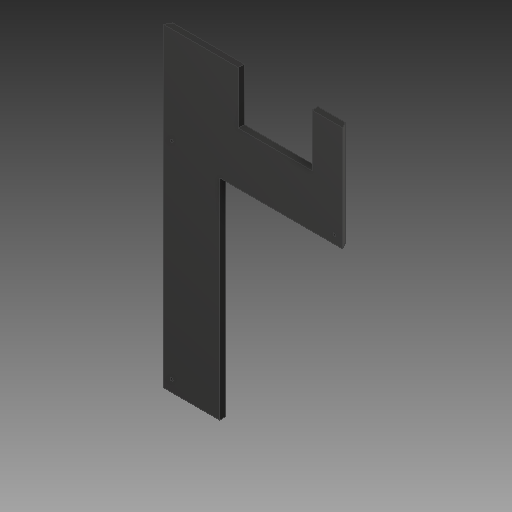
# Autodesk Inventor part: BA03
Saved by Autodesk Inventor 2017 (Build 210142000, 142)
## iProperties
Created: 2018-10-18
Part Number: BA03
Material: ABS Plastic
Document SubType Name: Modeling
Designer: Dell
Density: 1.06 g/cm^3
Appearance: Smooth - Black
Author: Dell
Autodesk Inventor part; units mm, degrees
ref_plane "YZ Plane" through (0, 0, 0) normal (1, 0, 0) x (0, 1, 0)
ref_plane "XZ Plane" through (0, 0, 0) normal (0, 1, 0) x (-1, 0, 0)
ref_plane "XY Plane" through (0, 0, 0) normal (0, 0, 1) x (1, 0, 0)
sketch "Sketch1" plane through (0, 0, 0) normal (0, 0, 1) x (1, 0, 0)
  line L0 (0, 0) -> (292.1, 0)
  line L1 (292.1, 0) -> (292.1, -177.8)
  line L2 (292.1, -177.8) -> (0, -177.8)
  line L3 (0, -177.8) -> (0, 0)
  dimension "d0" = 292.1
  dimension "d1" = 177.8
  constraints: 8 end point, 2 parallel, 1 horizontal, 1 perpendicular
  measures "d0" distance of L1.end L2.end
  measures "d1" distance of L0.end L1.end
extrude "Extrusion1" add sketch "Sketch1" along normal blind 10
sketch "Sketch2" plane through (0, 0, 0) normal (0, 1, 0) x (1, 0, 0)
  line L0 (292.1, -10) -> (0, -10) projected
  line L1 (0, -10) -> (-5.7735, -10)
  line L2 (-5.7735, -10) -> (0, 0)
  line L3 (0, 0) -> (0, -10) projected
  line L4 (0, 0) -> (0, -10) projected
  line L5 (0, -10) -> (0, 0)
  line L6 (292.1, -10) -> (297.8735, -10)
  line L7 (292.1, 0) -> (292.1, -10) projected
  line L8 (297.8735, -10) -> (292.1, 0)
  line L9 (292.1, 0) -> (292.1, -10)
  dimension "d4" = 30
  dimension "d5" = 60
  constraints: 12 end point, 2 collinear, 2 horizontal
  measures "d4" angle of L3 L2
  measures "d5" angle of L6 L8
extrude "Extrusion2" add sketch "Sketch2" against normal blind 177.8
sketch "Sketch3" plane through (0, 0, 10) normal (0, 0, 1) x (1, 0, 0)
  line L0 (46.05, -88.9) -> (246.05, -88.9)
  line L1 (246.05, -88.9) -> (246.05, 0)
  line L2 (246.05, 0) -> (46.05, 0)
  line L3 (46.05, 0) -> (46.05, -88.9)
  line L4 (-5.7735, 0) -> (297.8735, 0) projected
  line L5 (46.05, -88.9) -> (190.7027, -88.9)
  line L6 (121.05, 0) -> (46.05, 0)
  line L7 (46.05, 0) -> (46.05, -88.9)
  line L8 (246.05, 0) -> (171.05, 0)
  line L9 (121.05, -88.9) -> (246.05, -88.9)
  line L10 (246.05, -88.9) -> (246.05, 0)
  line L11 (46.05, 0) -> (121.05, 0)
  line L12 (121.05, 0) -> (121.05, -88.9)
  line L13 (121.05, -88.9) -> (46.05, -88.9)
  line L14 (46.05, -88.9) -> (46.05, 0)
  line L15 (246.05, 0) -> (246.05, 0)
  line L16 (246.05, 0) -> (246.05, -88.9)
  line L17 (246.05, -88.9) -> (246.05, -88.9)
  line L18 (246.05, -88.9) -> (246.05, 0)
  point P0 (0, 0)
  point P1 (146.05, 0)
  point P2 (246.05, -44.45)
  dimension "d8" = 200
  dimension "d9" = 88.9
  dimension "d14" = 75
  constraints: 36 end point, 7 parallel, 5 horizontal, 4 midpoint, 3 perpendicular, 3 point on line, 1 collinear
  measures "d8" distance of L1.end L2.end
  measures "d9" distance of L0.end L1.end
  measures "d14" distance between parallel lines of L3 L12
extrude "Extrusion3" cut sketch "Sketch3" against normal through all contours L12 L2 L1 L0
sketch "Sketch4" plane through (0, 0, 10) normal (0, 0, 1) x (1, 0, 0)
  line L0 (8.1265, -163.9) -> (283.9735, -163.9) construction
  line L1 (297.8735, -177.8) -> (-5.7735, -177.8) construction
  line L2 (297.8735, 0) -> (297.8735, -177.8) construction
  line L3 (-5.7735, 0) -> (-5.7735, -177.8) construction
  circle A0 centre (8.1265, -163.9) radius 2.5
  circle A1 centre (283.9735, -163.9) radius 2.5
  point P0 (0, 0)
  dimension "d16" = 13.9
  dimension "d17" = 13.9
  dimension "d18" = 13.9
  dimension "d19" = 5
  dimension "d20" = 5
  constraints: 2 centre point, 2 coincident, 2 end point, 1 horizontal
  measures "d16" distance between parallel lines of L1 L0
  measures "d17" distance from line of L2 L0.end
  measures "d18" distance from line of L3 L0.start
  measures "d19" diameter of A0
  measures "d20" diameter of A1
extrude "Extrusion4" cut sketch "Sketch4" against normal through all
sketch "Sketch5" plane through (0, 0, 10) normal (0, 0, 1) x (1, 0, 0)
  line L0 (297.8735, -177.8) -> (-5.7735, -177.8) projected
  line L1 (-5.7735, -177.8) -> (89.4765, -177.8)
  line L2 (89.4765, -177.8) -> (89.4765, -533.4)
  line L3 (89.4765, -533.4) -> (-5.7735, -533.4)
  line L4 (-5.7735, -533.4) -> (-5.7735, -177.8)
  point P0 (0, 0)
  dimension "d23" = 95.25
  dimension "d24" = 355.6
  constraints: 8 end point, 2 parallel, 1 horizontal, 1 perpendicular
  measures "d23" distance between parallel lines of L2 L4
  measures "d24" distance of L3.end L0.end
extrude "Extrusion5" add sketch "Sketch5" against normal blind 10
sketch "Sketch6" plane through (-5.7735, -177.8, 0) normal (0, 1, 0) x (1, 0, 0)
  line L0 (0, -10) -> (5.7735, 0) projected
  line L1 (0, 0) -> (5.7735, 0) projected
  line L2 (0, -10) -> (0, 0) projected
  point P0 (5.7735, 0)
extrude "Extrusion6" cut sketch "Sketch6" against normal through all
sketch "Sketch7" plane through (0, 0, 10) normal (0, 0, 1) x (1, 0, 0)
  circle A0 centre (8.1265, -514.35) radius 2.5
  line L0 (89.4765, -533.4) -> (0, -533.4) projected
  circle A1 centre (8.1265, -163.9) radius 2.5 projected
  point P0 (0, 0)
  dimension "d29" = 5
  dimension "d30" = 19.05
  constraints: 1 centre point, 1 vertical alignment
  measures "d29" diameter of A0
  measures "d30" distance from line of L0 A0.centre
extrude "Extrusion7" cut sketch "Sketch7" against normal through all contours A0
body "Solid1"
